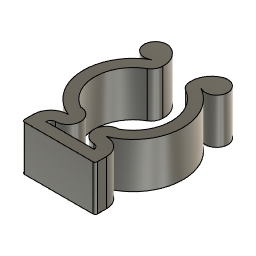
ETRIE DE FIXATION MECA PROJET 1 17-22 MM v1 v1 (Autodesk Fusion 360 design; units mm, degrees)
Autodesk Fusion 360 part; units mm, degrees
note: some values were not read from the file. Set by a fixed rule: which sketch regions a step uses.
sketch "Esquisse1" plane through (0, 0, 0) normal (0, 0, 1) x (1, 0, 0)
  line L0 (-7.589, -16.4847) -> (7.589, -16.4847)
  line L1 (8.089, -15.9847) -> (8.089, -13.9847)
  line L2 (-8.089, -13.9847) -> (-8.089, -15.9847)
  line L3 (0, 19.9726) -> (0, -22.061) construction
  line L4 (4.25, 7.3612) -> (6.75, 7.3612) construction
  line L5 (-4.25, 7.3612) -> (-1.75, 7.3612) construction
  arc A0 (-4.25, 7.3612) -> (-4.25, -7.3612) centre (0, 0) ccw
  arc A1 (4.25, -7.3612) -> (4.25, 7.3612) centre (0, 0) ccw
  arc A2 (-5.5, 9.5263) -> (-4.25, -10.1458) centre (0, 0) ccw
  arc A3 (4.25, -10.1458) -> (5.5, 9.5263) centre (0, 0) ccw
  arc A4 (-4.25, -10.1458) -> (-8.0889, -13.9847) centre (-4.25, -13.9847) ccw
  arc A5 (-4.25, -12.9304) -> (-4.25, -7.3612) centre (-4.25, -10.1458) ccw
  arc A6 (-4.25, -12.9304) -> (-5.3043, -13.9847) centre (-4.25, -13.9847) ccw
  arc A7 (8.0889, -13.9847) -> (4.25, -10.1458) centre (4.25, -13.9847) ccw
  arc A8 (4.25, -7.3612) -> (4.25, -12.9304) centre (4.25, -10.1458) ccw
  arc A9 (5.3043, -13.9847) -> (4.25, -12.9304) centre (4.25, -13.9847) ccw
  arc A10 (4.25, -10.1458) -> (5.5, 9.5263) centre (0, 0) ccw
  arc A11 (4.25, -7.3612) -> (4.25, 7.3612) centre (0, 0) ccw
  arc A12 (-4.25, 7.3612) -> (-3, 9.5263) centre (-5.5, 9.5263) ccw
  arc A13 (-5.7636, 13.9885) -> (-5.5, 9.5263) centre (-6.75, 11.6913) ccw
  arc A14 (-3, 9.5263) -> (-5.7636, 13.9885) centre (-7.5693, 9.7833) ccw
  arc A15 (5.5, 9.5263) -> (5.7636, 13.9885) centre (6.75, 11.6913) ccw
  arc A16 (5.7636, 13.9885) -> (3, 9.5263) centre (7.5693, 9.7833) ccw
  arc A17 (3, 9.5263) -> (4.25, 7.3612) centre (5.5, 9.5263) ccw
  arc A18 (4.25, -7.3612) -> (4.25, 7.3612) centre (0, 0) ccw
  arc A19 (4.25, -10.1458) -> (5.5, 9.5263) centre (0, 0) ccw
  arc A20 (8.0889, -13.9847) -> (4.25, -10.1458) centre (4.25, -13.9847) ccw
  arc A21 (4.25, -7.3612) -> (4.25, -12.9304) centre (4.25, -10.1458) ccw
  arc A22 (5.3043, -13.9847) -> (4.25, -12.9304) centre (4.25, -13.9847) ccw
  line L6 (-8.0889, -13.9847) -> (-8.089, -13.9847)
  line L7 (8.089, -13.9847) -> (8.0889, -13.9847)
  line L8 (5.3043, -13.9847) -> (-5.3043, -13.9847)
  line L9 (8.0889, -13.9847) -> (8.089, -13.9847)
  line L10 (-8.089, -13.9847) -> (-8.0889, -13.9847)
  line L11 (-5.3043, -13.9847) -> (5.3043, -13.9847)
  arc A23 (-8.089, -15.9847) -> (-7.589, -16.4847) centre (-7.589, -15.9847) ccw
  arc A24 (7.589, -16.4847) -> (8.089, -15.9847) centre (7.589, -15.9847) ccw
  point P0 (-8.089, -16.4847)
  dimension "d1" = 17
  dimension "d2" = 22
  dimension "d3" = 2.5
  dimension "d8" = 16.178
  dimension "d9" = 3.8389
  dimension "d11" = 8.5
  dimension "d12" = 8.089
  dimension "d13" = 0.5
  dimension "d14" = 0.5
  constraint coincident A0.centre A1.centre
  constraint concentric A0 A2
  constraint horizontal L0
  constraint vertical L1
  constraint horizontal L7
  constraint vertical L2
  constraint coincident A0.centre L3
  constraint horizontal L4
  constraint horizontal L5
  constraint coincident A1.start A0
  constraint concentric A0 A1
  constraint concentric A2 A3
  constraint coincident A2.end A4.start
  constraint coincident A4.end L7
  constraint concentric A4 A6
  constraint tangent A5 A6
  constraint symmetric L1.end L3 L2.start
  constraint symmetric L2.start L3 L1.end
  constraint symmetric L3 L5.start L4.start
  constraint symmetric L3 A2.start A3.end
  constraint symmetric L3 A0.end A1.start
  constraint symmetric L3 A0 A11
  constraint symmetric L3 A2 A10
  constraint symmetric L3 A2.end A3.start
  constraint symmetric L3 A4.end A7.start
  constraint symmetric L3 A4 A7
  constraint symmetric L3 A5 A8
  constraint symmetric L3 A5.start A8.end
  constraint symmetric L3 A6 A9
  constraint symmetric L3 A6.end A9.start
  constraint coincident A2.start A12.centre
  constraint tangent A0 A12
  constraint coincident A2.start A13
  constraint tangent A13 A14
  constraint symmetric L3 A0 A18
  constraint symmetric L3 A2 A19
  constraint symmetric L3 A4 A20
  constraint symmetric L3 A5 A21
  constraint symmetric L3 A6 A22
  constraint symmetric L3 A12 A17
  constraint symmetric L3 A13 A15
  constraint symmetric L3 A13.start A15.end
  constraint symmetric L3 A12.end A16.end
  constraint symmetric L3 A14 A16
  constraint collinear L6 L7
  constraint collinear L7 L8
  constraint collinear L9 L10
  constraint collinear L10 L11
  constraint coincident P0 L2
  constraint coincident P0 L0
  constraint tangent L2 A23
  constraint tangent L0 A23
  constraint tangent L1 A24
  constraint tangent L0 A24
  measures "d1" diameter of A0
  measures "d2" diameter of A2
  measures "d3" distance of P0 L2.start
  measures "d8" distance of L1 L2
  measures "d9" distance of A2.end L7
  measures "d11" distance of A2.end A3.start
  measures "d12" distance of L2 L3
  measures "d13" radius of A23
  measures "d14" radius of A24
extrude "Extrusion1" add sketch "Esquisse1" along normal blind 10
